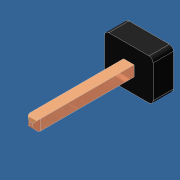
# Autodesk Inventor part: 2009_CTS_CopperPost
Saved by Autodesk Inventor 2012 (Build 160160000, 160)
## iProperties
Company: Team 801
Created: 2009-01-31
Part Number: 2009_CTS_CopperPost
Document SubType Name: Modeling
Designer: Jeffrey M
Density: 1 g/cm^3
Material: Default
Mass: 0.0123083 g
Surface Area: 0.445979 cm^2
Volume: 0.0123083 cm^3
Title: 2009_CTS_CopperPost
Author: Jeffrey M
Autodesk Inventor part; units mm, degrees
ref_plane "YZ Plane" through (0, 0, 0) normal (1, 0, 0) x (0, 1, 0)
ref_plane "XZ Plane" through (0, 0, 0) normal (0, 1, 0) x (-1, 0, 0)
ref_plane "XY Plane" through (0, 0, 0) normal (0, 0, 1) x (1, 0, 0)
sketch "Sketch1" plane through (0, 0, 0) normal (0, 0, 1) x (1, 0, 0)
  line L0 (-0.6632, 1.4381) -> (-3.6858, 1.4381)
  line L1 (-3.6858, 1.4381) -> (-3.6858, 3.9781)
  line L2 (-3.6858, 3.9781) -> (-0.6632, 3.9781)
  line L3 (-0.6632, 3.9781) -> (-0.6632, 1.4381)
  dimension "d0" = 3.0226
  dimension "d1" = 2.54
  constraints: 8 end point, 2 parallel, 1 horizontal, 1 perpendicular
  measures "d0" distance of L1.end L2.end
  measures "d1" distance of L2.end L0.start
extrude "Extrusion1" add sketch "Sketch1" along normal blind 1.27
sketch "Sketch2" plane through (0, 0, 1.27) normal (0, 0, 1) x (1, 0, 0)
  line L0 (-2.5047, 3.0383) -> (-1.8443, 3.0383)
  line L1 (-1.8443, 3.0383) -> (-1.8443, 2.3779)
  line L2 (-1.8443, 2.3779) -> (-2.5047, 2.3779)
  line L3 (-2.5047, 2.3779) -> (-2.5047, 3.0383)
  point P0 (-2.1745, 2.7081)
  dimension "d6" = 0.3302
  dimension "d7" = 0.3302
  dimension "d8" = 0.3302
  dimension "d9" = 0.3302
  constraints: 8 end point, 2 parallel, 1 horizontal, 1 perpendicular
  measures "d6" distance from line of point (-2.175, 2.708) L3
  measures "d7" distance from line of point (-2.175, 2.708) L1
  measures "d8" distance from line of L0 point (-2.175, 2.708)
  measures "d9" distance from line of L2 point (-2.175, 2.708)
extrude "Extrusion2" add sketch "Sketch2" along normal blind 6.096
fillet "Fillet1" radius 0.254 4 edges at (-2.1745, 2.3779, 7.366) (-1.8443, 2.7081, 7.366) (-2.1745, 3.0383, 7.366) (-2.5047, 2.7081, 7.366)
fillet "Fillet2" radius 0.254 4 edges at (-3.6858, 1.4381, 0.635) (-0.6632, 1.4381, 0.635) (-0.6632, 3.9781, 0.635) (-3.6858, 3.9781, 0.635)
equation "\"d7\" = d6"
equation "\"d8\" = d6"
equation "\"d9\" = d8"
body "Solid1"
